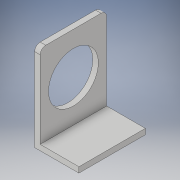
# Autodesk Inventor part: ARM_011_BearingMount
Saved by Autodesk Inventor 2018.3 (Build 223284000, 284)
## iProperties
Created: 2020-01-31
Part Number: ARM_011_BearingMount
Material: Generic
Document SubType Name: Modeling
Designer: 21vogecale
Density: 1 g/cm^3
Appearance: Default
Author: 21vogecale
Autodesk Inventor part; units mm, degrees
ref_plane "YZ Plane" through (0, 0, 0) normal (1, 0, 0) x (0, 1, 0)
ref_plane "XZ Plane" through (0, 0, 0) normal (0, 1, 0) x (-1, 0, 0)
ref_plane "XY Plane" through (0, 0, 0) normal (0, 0, 1) x (1, 0, 0)
sketch "Sketch1" plane through (0, 0, 0) normal (0, 1, 0) x (-1, 0, 0)
  line L0 (-15.875, 28.575) -> (9.525, 28.575)
  line L1 (9.525, 28.575) -> (9.525, -9.525)
  line L2 (9.525, -9.525) -> (-15.875, -9.525)
  line L3 (-15.875, -9.525) -> (-15.875, 28.575)
  point P0 (0, 0)
  dimension "d0" = 38.1
  dimension "d1" = 25.4
  dimension "d2" = 9.525
  dimension "d3" = 9.525
  constraints: 8 end point, 2 parallel, 1 horizontal, 1 perpendicular
  measures "d0" distance of L0.end L1.end
  measures "d1" distance of L1.end L2.end
  measures "d2" distance from line of point (0, 0) L1
  measures "d3" distance from line of L2 point (0, 0)
extrude "Extrusion1" add sketch "Sketch1" along normal blind 3.175
sketch "Sketch4" plane through (-9.525, 0, -9.525) normal (-1, 0, 0) x (0, 0, 1)
  circle A0 centre (19.05, 27.0002) radius 14.2875
  line L0 (38.1, 0) -> (38.1, 3.175) projected
  line L1 (38.1, 3.175) -> (0, 3.175) projected
  line L2 (0, 0) -> (38.1, 0) projected
  line L3 (0, 0) -> (38.1, 0)
  line L4 (38.1, 0) -> (38.1, 50.8)
  line L5 (38.1, 50.8) -> (0, 50.8)
  line L6 (0, 50.8) -> (0, 0)
  point P0 (9.525, 0)
  dimension "d11" = 19.05
  dimension "d12" = 28.575
  dimension "d14" = 50.8
  dimension "d18" = 27.0002
  dimension "d19" = 38.1
  constraints: 8 end point, 2 parallel, 1 centre point, 1 horizontal, 1 perpendicular
  measures "d11" distance from line of L0 A0.centre
  measures "d12" diameter of A0
  measures "d14" distance between parallel lines of L2 L5
  measures "d18" distance from line of L2 A0.centre
  measures "d19" distance of L4.end L5.end
extrude "Extrusion2" add sketch "Sketch4" against normal blind 3.175
fillet "Fillet1" radius 3.175 2 edges at (-7.9375, 50.8, 28.575) (-7.9375, 50.8, -9.525)
body "Solid1"
